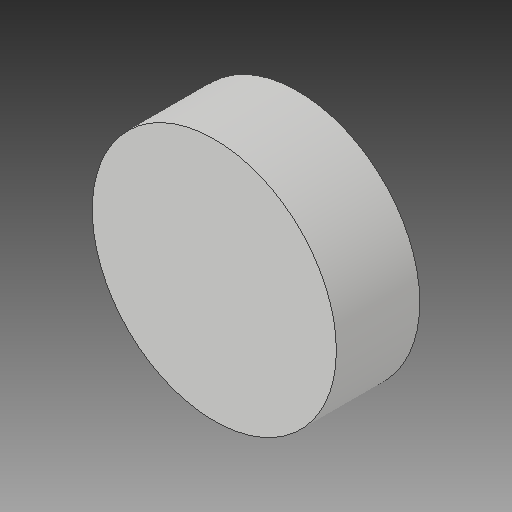
# Autodesk Inventor part: ThumbScrew
Saved by Autodesk Inventor 2018 (Build 220112000, 112)
## iProperties
Created: 2018-05-20
Part Number: ThumbScrew
Material: Generic
Document SubType Name: Modeling
Designer: reide
Density: 1 g/cm^3
Appearance: Default
Author: reide
Autodesk Inventor part; units mm, degrees
ref_plane "YZ Plane" through (0, 0, 0) normal (1, 0, 0) x (0, 1, 0)
ref_plane "XZ Plane" through (0, 0, 0) normal (0, 1, 0) x (-1, 0, 0)
ref_plane "XY Plane" through (0, 0, 0) normal (0, 0, 1) x (1, 0, 0)
sketch "Sketch1" plane through (0, 0, 0) normal (0, 0, 1) x (1, 0, 0)
  circle A0 centre (-68.6105, -28.321) radius 1.63 projected
  circle A1 centre (-68.6105, -28.321) radius 2.875
  circle A2 centre (-68.6105, -28.321) radius 6
  point P0 (0, 0)
  dimension "d0" = 5.75
  dimension "d1" = 12
  constraints: 2 centre point, 2 coincident
  measures "d0" diameter of A1
  measures "d1" diameter of A2
extrude "Extrusion1" add sketch "Sketch1" along normal blind 3.1 contours A2
sketch "Sketch2" plane through (-68.6105, -28.321, 3.1) normal (0, 0, 1) x (1, 0, 0)
  circle A0 centre (0, 0) radius 2.875 projected
  circle A1 centre (0, 0) radius 6 projected
  point P0 (68.6105, 28.321)
extrude "Extrusion2" add sketch "Sketch2" along normal blind 1 contours A0 | A1
body "Solid1"
